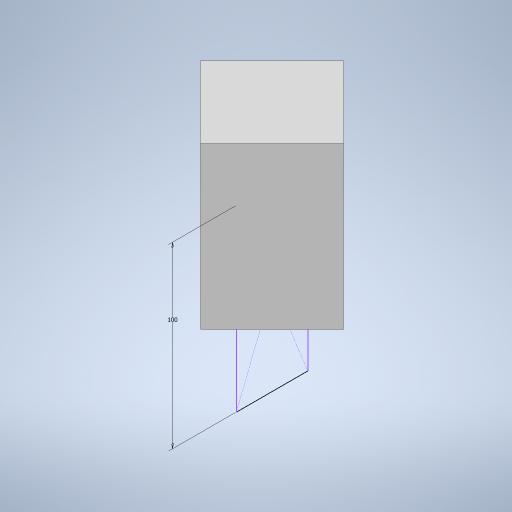
# Autodesk Inventor part: Деталь1
Saved by Autodesk Inventor 2023.2 (Build 272271030, 271C)
## iProperties
Created: 2023-09-29
Part Number: Деталь1
Material: Типовые
Document SubType Name: Modeling
Designer: User
Density: 1 g/cm^3
Appearance: По умолчанию
Author: User
Autodesk Inventor part; units mm, degrees
ref_plane "YZ Plane" through (0, 0, 0) normal (1, 0, 0) x (0, 1, 0)
ref_plane "XZ Plane" through (0, 0, 0) normal (0, 1, 0) x (-1, 0, 0)
ref_plane "XY Plane" through (0, 0, 0) normal (0, 0, 1) x (1, 0, 0)
sketch "Эскиз4" plane through (0, 0, 0) normal (0, 1, 0) x (-1, 0, 0)
  line L0 (-40, 0) -> (0, 40)
  line L1 (0, 40) -> (40, 0)
  line L2 (40, 0) -> (0, -40)
  line L3 (0, -40) -> (-40, 0)
  point P0 (0, 0)
  point P1 (0, 0)
  constraints: 8 end point, 9 other
extrude "Выдавливание2" add sketch "Эскиз4" along normal blind 90
sketch "Эскиз5" plane through (0, 0, 0) normal (1, 0, 0) x (0, 1, 0)
  line L0 (50, -19.8959) -> (-50, -19.8959)
  line L1 (-50, -19.8959) -> (-50, 19.8959)
  line L2 (-50, 19.8959) -> (50, 19.8959)
  line L3 (50, 19.8959) -> (50, -19.8959)
  line L4 (0, 0) -> (0, 40) projected
  line L5 (50, -19.8959) -> (-50, 19.8959) construction
  line L6 (-50, -19.8959) -> (50, 19.8959) construction
  dimension "d8" = 100
  constraints: 12 end point, 2 midpoint, 2 parallel, 1 horizontal, 1 perpendicular
  measures "d8" distance of L1.end L2.end
